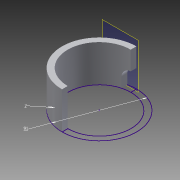
# Autodesk Inventor part: BurkolatPVCszenzor
Saved by Autodesk Inventor 2015 SP1 (Build 190203100, 203)
## iProperties
Created: 2014-11-14
Part Number: BurkolatPVCszenzor
Material: PVC-Piping
Document SubType Name: Modeling
Designer: laca
Density: 1.4 g/cm^3
Appearance: Smooth - White
Mass: 56.2258 g
Surface Area: 139.252 cm^2
Volume: 40.1613 cm^3
KulsoAtmeroPVCcso: 91.000 mm
PVCfalVastagsag: 7.000 mm
d2: 45.000 mm
d3: 0.00 deg
KisFogaskerekBesulyesztes: 12.000 mm
Author: laca
Autodesk Inventor part; units mm, degrees
ref_plane "YZ Plane" through (0, 0, 0) normal (1, 0, 0) x (0, 1, 0)
ref_plane "XZ Plane" through (0, 0, 0) normal (0, 1, 0) x (-1, 0, 0)
ref_plane "XY Plane" through (0, 0, 0) normal (0, 0, 1) x (1, 0, 0)
sketch "Sketch1" plane through (0, 0, 0) normal (0, 1, 0) x (-1, 0, 0)
  circle A0 centre (0, 0) radius 45.5
  circle A1 centre (0, 0) radius 38.5
  line L0 (0, 45.5) -> (0, 38.5)
  line L1 (0, -38.5) -> (0, -45.5)
  dimension "KulsoAtmeroPVCcso" = 91
  dimension "PVCfalVastagsag" = 7
  constraints: 4 end point, 4 point on circle, 2 centre point, 2 coincident, 2 line through centre, 2 vertical
  measures "KulsoAtmeroPVCcso" diameter of A0
  measures "PVCfalVastagsag" radial gap between concentric circles of A0 A1
extrude "Extrusion1" add sketch "Sketch1" along normal blind 45 contours A0 L1 A1 L0 picked at (28.7594, -28.7594)
ref_plane "Work Plane1" through (0, 0, -45.5) normal (0, 0, -1) x (-1, 0, 0)
sketch "Sketch2" plane through (0, 0, -45.5) normal (0, 0, -1) x (-1, 0, 0)
  arc A0 (10, 12) -> (0, 2) centre (0, 12) ccw
  line L0 (10, 12) -> (10, 0)
  line L1 (0, 0) -> (38.5, 0) projected
  line L2 (10, 0) -> (0, 0)
  line L3 (0, 0) -> (0, 12)
  line L4 (0, 0) -> (0, 45) projected
  dimension "d4" = 20
  dimension "KisFogaskerekBesulyesztes" = 12
  constraints: 6 end point, 2 point on circle, 2 point on line, 1 centre point, 1 collinear, 1 horizontal, 1 vertical, 1 vertical alignment
  measures "d4" diameter of A0
  measures "KisFogaskerekBesulyesztes" distance of L1.start L3.end
extrude "Extrusion2" cut sketch "Sketch2" against normal blind 50
body "Solid1"
